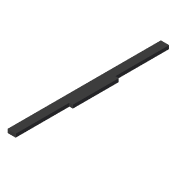
# Autodesk Inventor part: Lateral Potentiometers short
Saved by Autodesk Inventor 2020 (Build 240168000, 168)
## iProperties
Created: 2020-11-07
Part Number: Lateral Potentiometers short
Material: Generic
Document SubType Name: Modeling
Designer: ferrerx
Density: 1 g/cm^3
Appearance: Default
Author: ferrerx
Autodesk Inventor part; units mm, degrees
ref_plane "YZ Plane" through (0, 0, 0) normal (1, 0, 0) x (0, 1, 0)
ref_plane "XZ Plane" through (0, 0, 0) normal (0, 1, 0) x (-1, 0, 0)
ref_plane "XY Plane" through (0, 0, 0) normal (0, 0, 1) x (1, 0, 0)
sketch "Sketch1" plane through (0, 0, 0) normal (0, 1, 0) x (-1, 0, 0)
  line L0 (0, 0) -> (7, 0)
  line L1 (7, 0) -> (7, -134)
  line L2 (7, -134) -> (0, -134)
  line L3 (0, -134) -> (0, 0)
  line L4 (0, -47) -> (-3, -47)
  line L5 (-3, -47) -> (-3, -87)
  line L6 (-3, -87) -> (0, -87)
  line L7 (0, -87) -> (0, -47)
  line L8 (7, -67) -> (0, -67) construction
  line L9 (-3, -67) -> (0, -67) construction
  point P0 (0, -87)
  dimension "d0" = 134
  dimension "d1" = 3
  dimension "d2" = 40
  dimension "d3" = 7
  constraints: 20 end point, 4 midpoint, 4 parallel, 2 horizontal, 2 perpendicular, 1 collinear, 1 point on line
  measures "d0" distance of L2.end L0.start
  measures "d1" distance of L5.end L6.end
  measures "d2" distance of L4.end L5.end
  measures "d3" distance of L1.end L2.end
extrude "Extrusion1" add sketch "Sketch1" along normal blind 3
body "Solid1"
